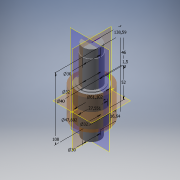
# Autodesk Inventor part: Вал переходный
Saved by Autodesk Inventor 2018 (Build 220112000, 112)
## iProperties
Created: 2018-03-24
Part Number: Вал переходный
Material: Типовые
Document SubType Name: Modeling
Designer: kriku
Density: 1 g/cm^3
Appearance: По умолчанию
Mass: 159.882 g
Surface Area: 198.862 cm^2
Volume: 159.882 cm^3
Author: kriku
Autodesk Inventor part; units mm, degrees
sketch "Эскиз1" plane through (0, 0, 0) normal (1, 0, 0) x (0, 1, 0)
  line L0 (15, 87.45) -> (15, 73.5)
  line L1 (15, 73.5) -> (16, 73.5)
  line L2 (16, 73.5) -> (16, 27.5)
  line L3 (16, 27.5) -> (20, 27.5)
  line L4 (20, 27.5) -> (20, 26)
  line L5 (20, 26) -> (23.801, 26)
  line L6 (23.801, 26) -> (23.801, -26)
  line L7 (23.801, -26) -> (16, -26)
  line L8 (16, -34.5) -> (15, -34.5)
  line L9 (15, -34.5) -> (15, -51.1401)
  line L10 (15, -51.1401) -> (0, -51.1401)
  line L11 (15, 87.45) -> (0, 87.45)
  line L12 (0, 87.45) -> (0, -51.1401)
  line L13 (27.551, 26) -> (27.551, -26)
  line L14 (30.551, 26) -> (30.551, -26)
  line L15 (30.551, 26) -> (23.801, 26)
  line L16 (30.551, -26) -> (23.801, -26)
  line L17 (16, -26) -> (16, -34.5)
  line L18 (-6.1102, 0) -> (36.6612, 0) projected
  line L19 (0, 115.168) -> (0, -78.8581) projected
  point P0 (0, 0)
  dimension "d0" = 40
  dimension "d1" = 32
  dimension "d2" = 30
  dimension "d3" = 30
  dimension "d4" = 47.602
  dimension "d5" = 27.551
  dimension "d6" = 61.102
  dimension "d7" = 108
  dimension "d8" = 52
  dimension "d9" = 1.5
  dimension "d10" = 46
  dimension "d13" = 32
  dimension "d14" = 16.6401
  dimension "d15" = 138.5901
  constraints: 36 end point, 9 perpendicular, 4 horizontal, 3 parallel, 3 vertical, 1 horizontal alignment, 1 point on line, 1 other
  measures "d0" diameter of L4 L12
  measures "d1" diameter of L2 L12
  measures "d2" diameter of L0 L12
  measures "d3" diameter of L9 L12
  measures "d4" diameter of L6 L12
  measures "d5" distance between parallel lines of L12 L13
  measures "d6" diameter of L14 L12
  measures "d7" distance between parallel lines of L8 L1
  measures "d8" distance of L14.start L14.end
  measures "d9" distance of L3.end L4.end
  measures "d10" distance of L1.end L2.end
  measures "d13" diameter of L17 L12
  measures "d14" distance of L8.end L9.end
  measures "d15" distance between parallel lines of L11 L10
surface revolve "ВращПврх1" sketch "Эскиз1" angle 360 about axis through (0, 0, 87.45) along (0, 0, -1) shown yes curves L15 L14 L16
revolve "Вращение1" add sketch "Эскиз1" angle 360 about axis through (0, 0, 87.45) along (0, 0, -1) contours L0 L1 L2 L3 L4 L5 L6 L18 L12 L11 | L18 L6 L7 L17 L8 L9 L10 L12
body "SRF1"
